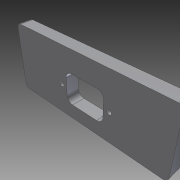
# Autodesk Inventor part: front cover
Saved by Autodesk Inventor 2012 (Build 160160000, 160)
## iProperties
Created: 2017-04-27
Part Number: front cover
Material: Default
Document SubType Name: Modeling
Designer: Brandon
Density: 1 g/cm^3
Author: Brandon
Autodesk Inventor part; units mm, degrees
ref_plane "YZ Plane" through (0, 0, 0) normal (1, 0, 0) x (0, 1, 0)
ref_plane "XZ Plane" through (0, 0, 0) normal (0, 1, 0) x (-1, 0, 0)
ref_plane "XY Plane" through (0, 0, 0) normal (0, 0, 1) x (1, 0, 0)
sketch "Sketch1" plane through (0, 0, 0) normal (0, 0, 1) x (1, 0, 0)
  line L0 (-62.4, 25.45) -> (62.4, 25.45)
  line L1 (62.4, 25.45) -> (62.4, -25.45)
  line L2 (62.4, -25.45) -> (-62.4, -25.45)
  line L3 (-62.4, -25.45) -> (-62.4, 25.45)
  point P0 (0, 0)
  dimension "d0" = 124.8
  dimension "d1" = 50.9
  dimension "d2" = 62.4
  dimension "d3" = 25.45
  constraints: 8 end point, 2 parallel, 1 horizontal, 1 perpendicular
  measures "d0" distance of L1.end L2.end
  measures "d1" distance of L0.end L1.end
  measures "d2" distance from line of point (0, 0) L3
  measures "d3" distance from line of L0 point (0, 0)
extrude "Extrusion1" add sketch "Sketch1" along normal blind 10.0076
fillet "Fillet1" radius 3.175 1 edges at (-62.4, 25.45, 5.0038)
fillet "Fillet2" radius 3.175 3 edges at (62.4, 25.45, 5.0038) (62.4, -25.45, 5.0038) (-62.4, -25.45, 5.0038)
sketch "Sketch6" plane through (0, 0, 10.0076) normal (0, 0, 1) x (1, 0, 0)
  arc A0 (10.55, -12.337) -> (15.55, -7.337) centre (10.55, -7.337) ccw projected
  line L0 (15.55, -7.337) -> (15.55, 5.963) projected
  arc A1 (15.55, 5.963) -> (10.55, 10.963) centre (10.55, 5.963) ccw projected
  line L1 (10.55, 10.963) -> (-10.55, 10.963) projected
  arc A2 (-10.55, 10.963) -> (-15.55, 5.963) centre (-10.55, 5.963) ccw projected
  line L2 (-15.55, 5.963) -> (-15.55, -7.337) projected
  arc A3 (-15.55, -7.337) -> (-10.55, -12.337) centre (-10.55, -7.337) ccw projected
  line L3 (-10.55, -12.337) -> (10.55, -12.337) projected
  circle A4 centre (-20, -0.687) radius 1.8 projected
  circle A5 centre (20, -0.687) radius 1.8 projected
  point P0 (0, 0)
extrude "Extrusion7" cut sketch "Sketch6" against normal up to surface (10.0076 mm away)
equation "\"d2\" = 0.5 * d0"
equation "\"d3\" = 0.5 * d1"
body "Solid1"
